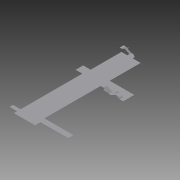
# Autodesk Inventor part: LabVIEWM0.5
Saved by Autodesk Inventor 2013 SP2 (Build 170200200, 200)
## iProperties
Created: 2014-11-17
Part Number: LabVIEWM0.5
Material: 常规
Document SubType Name: Modeling
Designer: 振胜
Density: 1 g/cm^3
Author: 振胜
Autodesk Inventor part; units mm, degrees
ref_plane "YZ Plane" through (0, 0, 0) normal (1, 0, 0) x (0, 1, 0)
sketch "DOOR" plane through (0, 0, 0) normal (0, 0, 1) x (1, 0, 0)
  line L0 (72.1652, -32.5468) -> (92.1652, -32.5468)
  line L1 (92.1652, -32.5468) -> (92.1652, -42.5468)
  line L2 (92.1652, -42.5468) -> (72.1652, -42.5468)
  line L3 (72.1652, -42.5468) -> (72.1652, -32.5468)
  line L4 (72.1652, -37.5468) -> (92.1652, -37.5468) construction
  dimension "d217" = 10
  dimension "d219" = 20
  measures "d217" distance between parallel lines of L2 L0
  measures "d219" distance between parallel lines of L1 L3
sketch "DOOR2" plane through (0, 0, 0) normal (0, 0, 1) x (1, 0, 0)
  line L0 (57.8646, 97.8913) -> (77.8646, 97.8913)
  line L1 (77.8646, 97.8913) -> (77.8646, 87.8913)
  line L2 (77.8646, 87.8913) -> (57.8646, 87.8913)
  line L3 (57.8646, 87.8913) -> (57.8646, 97.8913)
  line L4 (57.8646, 92.8913) -> (77.8646, 92.8913) construction
  dimension "d227" = 10
  dimension "d229" = 20
  measures "d227" distance between parallel lines of L2 L0
  measures "d229" distance between parallel lines of L1 L3
ref_plane "工作平面1" through (0, 0, 0) normal (0, 0, 1) x (1, 0, 0)
sketch "草图1" plane through (0, 0, 0) normal (0, 0, 1) x (1, 0, 0)
  line L0 (0, 0) -> (60, 0)
  line L1 (60, 0) -> (60, -1169.8)
  line L2 (60, -1169.8) -> (0, -1169.8)
  line L3 (0, -1169.8) -> (0, 0)
  line L4 (0, -80.6) -> (60, -80.6)
  line L5 (0, -191.9) -> (60, -191.9)
  line L6 (0, -276.5) -> (60, -276.5)
  line L7 (0, -335.9) -> (60, -335.9)
  line L8 (0, -420.6) -> (60, -420.6)
  line L9 (0, -550.6) -> (60, -550.6)
  line L10 (0, -677.8) -> (60, -677.8)
  line L11 (0, -782.9) -> (60, -782.9)
  line L12 (0, -839.5) -> (60, -839.5)
  line L13 (0, -923.6) -> (60, -923.6)
  line L14 (0, -1007.7) -> (60, -1007.7)
  line L15 (0, -1091.2) -> (60, -1091.2)
  line L16 (60, 0) -> (118.4, 0)
  line L17 (118.4, 0) -> (118.4, -23.7)
  line L18 (118.4, -23.7) -> (83.4, -23.7)
  line L19 (83.4, -23.7) -> (83.4, -79.7)
  line L20 (83.4, -79.7) -> (118.4, -79.7)
  line L21 (118.4, -79.7) -> (118.4, -137.6)
  line L22 (118.4, -137.6) -> (83.4, -137.6)
  line L23 (83.4, -137.6) -> (83.4, -276.5)
  line L24 (83.4, -276.5) -> (142.9, -276.5)
  line L25 (142.9, -276.5) -> (142.9, -379.5)
  line L26 (83.4, -276.5) -> (83.4, -379.5)
  line L27 (83.4, -379.5) -> (142.9, -379.5)
  line L28 (142.9, -379.5) -> (142.9, -463)
  line L29 (142.9, -463) -> (83.4, -463)
  line L30 (83.4, -463) -> (83.4, -379.5)
  line L31 (142.9, -463) -> (142.9, -566.2)
  line L32 (142.9, -566.2) -> (83.4, -566.2)
  line L33 (83.4, -566.2) -> (83.4, -463)
  line L34 (142.9, -566.2) -> (146.7, -566.2)
  line L35 (146.7, -566.2) -> (146.7, -616.2)
  line L36 (146.7, -616.2) -> (192.5, -616.2)
  line L37 (192.5, -616.2) -> (192.5, -673.2)
  line L38 (192.5, -616.2) -> (342.5, -616.2)
  line L39 (342.5, -616.2) -> (342.5, -673.2)
  line L40 (342.5, -673.2) -> (143.4, -673.2)
  line L41 (143.4, -673.2) -> (83.4, -673.2)
  line L42 (83.4, -673.2) -> (83.4, -1092.3)
  line L43 (83.4, -1092.3) -> (143.4, -1092.3)
  line L44 (143.4, -1092.3) -> (143.4, -673.2)
  line L45 (83.4, -754.3) -> (143.4, -754.3)
  line L46 (143.4, -837.8) -> (83.4, -837.8)
  line L47 (83.4, -893.6) -> (143.4, -893.6)
  line L48 (143.4, -978.3) -> (83.4, -978.3)
  line L49 (60, -1169.8) -> (188.1, -1169.8)
  line L50 (188.1, -1169.8) -> (188.1, -1092.3)
  line L51 (188.1, -1092.3) -> (143.4, -1092.3)
  line L52 (83.4, -1092.3) -> (83.4, -1117.3)
  line L53 (83.4, -1117.3) -> (188.1, -1117.3)
  line L54 (98.6, -1092.3) -> (98.6, -1117.3)
  line L55 (114.5, -1092.3) -> (114.5, -1117.3)
  line L56 (143.4, -1092.3) -> (143.4, -1117.3)
  line L57 (166.2, -1092.3) -> (166.2, -1117.3)
  line L58 (188.1, -1163.6) -> (336, -1163.6)
  line L59 (188.1, -1137.1) -> (336, -1137.1)
  line L60 (336, -1137.1) -> (336, -1163.6)
  line L61 (342.5, -616.2) -> (398.5, -616.2)
  line L62 (342.5, -673.2) -> (393, -673.2)
  line L63 (393, -673.2) -> (393, -1136.7)
  line L64 (393, -1136.7) -> (393, -1141.7)
  line L65 (393, -1136.7) -> (336, -1137.1)
  line L66 (336, -1163.6) -> (393, -1163.6)
  line L67 (393, -1163.6) -> (393, -1158.6)
  line L68 (393, -1163.6) -> (393, -1188.1)
  line L69 (393, -1188.1) -> (417, -1188.1)
  line L70 (417, -1188.1) -> (553.5, -1188.1)
  line L71 (542.5, -1023) -> (542.5, -911)
  line L72 (542.5, -911) -> (542.5, -800.2)
  line L73 (542.5, -800.2) -> (542.5, -673.6)
  line L74 (398.5, -499.2) -> (398.5, -384.2)
  line L75 (398.5, -616.2) -> (398.5, -499.2)
  line L76 (398.5, -616.2) -> (458.5, -616.2)
  line L77 (458.5, -616.2) -> (458.5, -384.2)
  line L78 (458.5, -384.2) -> (398.5, -384.2)
  line L79 (398.5, -499.2) -> (458.5, -499.2)
  line L80 (398.5, -441.7) -> (458.5, -441.7)
  line L81 (458.5, -384.2) -> (458.5, -354.2)
  line L82 (458.5, -354.2) -> (482.5, -369.2)
  line L83 (482.5, -369.2) -> (482.5, -384.2)
  line L84 (482.5, -384.2) -> (542.5, -384.2)
  line L85 (542.5, -384.2) -> (542.5, -413.6)
  line L86 (542.5, -413.6) -> (542.5, -443.7)
  line L87 (542.5, -443.7) -> (542.5, -498.7)
  line L88 (542.5, -498.7) -> (542.5, -616.2)
  line L89 (542.5, -413.6) -> (501.5, -413.6)
  line L90 (542.5, -443.7) -> (482.5, -443.7)
  line L91 (542.5, -616.2) -> (482.5, -616.2)
  line L92 (542.5, -498.7) -> (482.5, -498.7)
  line L93 (482.5, -410.1) -> (501.5, -410.1)
  line L94 (501.5, -410.1) -> (501.5, -423.1)
  line L95 (501.5, -423.1) -> (482.5, -423.1)
  line L96 (482.5, -384.2) -> (482.5, -410.1)
  line L97 (482.5, -423.1) -> (482.5, -616.2)
  line L98 (542.5, -616.2) -> (727.5, -616.2)
  line L99 (727.5, -616.2) -> (727.5, -673.6)
  line L100 (727.5, -673.6) -> (542.5, -673.6)
  line L101 (578, -673.6) -> (578, -726.6)
  line L102 (578, -726.6) -> (605, -726.6)
  line L103 (605, -726.6) -> (605, -673.6)
  line L104 (727.5, -673.6) -> (727.5, -726.6)
  line L105 (727.5, -726.6) -> (700.5, -726.6)
  line L106 (700.5, -726.6) -> (700.5, -673.6)
  line L107 (442.5, -384.2) -> (442.5, -354.2)
  line L108 (442.5, -354.2) -> (458.5, -354.2)
  line L109 (398.5, -384.2) -> (384.5, -384.2)
  line L110 (384.5, -384.2) -> (384.5, -354.2)
  line L111 (384.5, -354.2) -> (400.5, -354.2)
  line L112 (400.5, -354.2) -> (400.5, -384.2)
  line L113 (458.5, -673.3753) -> (458.5, -1136.7)
  line L114 (482.5, -673.4395) -> (482.5, -1136.7)
  line L115 (542.5, -673.6) -> (482.5, -673.4395)
  line L116 (458.5, -673.3753) -> (393, -673.2)
  line L117 (458.5, -673.3753) -> (483.6773, -673.4426) construction
  line L118 (393, -1136.7) -> (458.5, -1136.7)
  line L119 (482.5, -1136.7) -> (535.5, -1136.7)
  line L120 (458.5, -1136.7) -> (482.5, -1136.7) construction
  line L121 (542.5, -1136.7) -> (542.5, -1106.6) construction
  line L122 (553.5, -1188.1) -> (553.5, -1147.6)
  line L123 (553.5, -1147.6) -> (761.5, -1147.6)
  line L124 (761.5, -1147.6) -> (761.5, -1106.6)
  line L125 (761.5, -1106.6) -> (542.5, -1106.6)
  line L126 (535.5, -1106.6) -> (535.5, -1136.7)
  line L127 (542.5, -1106.6) -> (542.5, -1023)
  line L128 (535.5, -1136.7) -> (542.5, -1136.7) construction
  line L129 (542.5, -1106.6) -> (535.5, -1106.6)
  line L130 (542.5, -800.2) -> (482.5, -800.2)
  line L131 (542.5, -911) -> (482.5, -911)
  line L132 (542.5, -1023) -> (482.5, -1023)
  line L133 (458.5, -800.2) -> (393, -800.2)
  line L134 (482.5, -800.2) -> (458.5, -800.2) construction
  line L135 (458.5, -911) -> (393, -911)
  line L136 (482.5, -911) -> (458.5, -911) construction
  line L137 (458.5, -1023) -> (393, -1023)
  line L138 (482.5, -1023) -> (458.5, -1023) construction
  dimension "d1" = 60
  dimension "d2" = 80.6
  dimension "d3" = 111.3
  dimension "d4" = 84.6
  dimension "d5" = 59.4
  dimension "d6" = 84.7
  dimension "d7" = 130
  dimension "d8" = 127.2
  dimension "d9" = 105.1
  dimension "d10" = 56.6
  dimension "d11" = 84.1
  dimension "d12" = 84.1
  dimension "d13" = 83.5
  dimension "d14" = 78.6
  dimension "d15" = 58.4
  dimension "d16" = 23.7
  dimension "d17" = 35
  dimension "d18" = 56
  dimension "d19" = 57.9
  dimension "d20" = 35
  dimension "d21" = 138.9
  dimension "d22" = 59.5
  dimension "d23" = 103
  dimension "d24" = 83.5
  dimension "d25" = 103.2
  dimension "d26" = 59.5
  dimension "d27" = 3.8
  dimension "d28" = 50
  dimension "d29" = 45.8
  dimension "d30" = 57
  dimension "d31" = 150
  dimension "d32" = 57
  dimension "d33" = 199.1
  dimension "d34" = 60
  dimension "d36" = 81.1
  dimension "d37" = 83.5
  dimension "d38" = 55.8
  dimension "d39" = 84.7
  dimension "d40" = 114
  dimension "d41" = 128.1
  dimension "d42" = 25
  dimension "d43" = 15.2
  dimension "d44" = 15.9
  dimension "d45" = 28.9
  dimension "d46" = 22.8
  dimension "d47" = 21.9
  dimension "d48" = 147.9
  dimension "d49" = 6.2
  dimension "d50" = 26.5
  dimension "d51" = 56
  dimension "d52" = 50.5
  dimension "d53" = 463.5
  dimension "d54" = 5
  dimension "d55" = 5
  dimension "d56" = 24.5
  dimension "d57" = 24
  dimension "d58" = 136.5
  dimension "d60" = 112
  dimension "d61" = 110.8
  dimension "d62" = 126.6
  dimension "d64" = 117
  dimension "d65" = 115
  dimension "d66" = 60
  dimension "d67" = 30
  constraints: 274 end point, 81 perpendicular, 42 point on line, 25 parallel, 18 horizontal, 15 collinear, 4 vertical, 1 horizontal alignment, 1 midpoint, 1 vertical alignment, 30 other
  measures "d1" distance of L0.start L0.end
  measures "d2" distance between parallel lines of L4 L0
  measures "d3" distance between parallel lines of L5 L4
  measures "d4" distance between parallel lines of L6 L5
  measures "d5" distance between parallel lines of L7 L6
  measures "d6" distance between parallel lines of L8 L7
  measures "d7" distance between parallel lines of L9 L8
  measures "d8" distance between parallel lines of L10 L9
  measures "d9" distance between parallel lines of L11 L10
  measures "d10" distance between parallel lines of L12 L11
  measures "d11" distance between parallel lines of L13 L12
  measures "d12" distance between parallel lines of L14 L13
  measures "d13" distance between parallel lines of L15 L14
  measures "d14" distance between parallel lines of L2 L15
  measures "d15" distance of L0.end L16.end
  measures "d16" distance of L16.end L17.end
  measures "d17" distance of L17.end L18.end
  measures "d18" distance of L18.end L19.end
  measures "d19" distance of L20.end L21.end
  measures "d20" distance of L21.end L22.end
  measures "d21" distance of L22.end L23.end
  measures "d22" distance of L23.end L24.end
  measures "d23" distance of L24.end L25.end
  measures "d24" distance of L25.end L28.end
  measures "d25" distance of L28.end L31.end
  measures "d26" distance of L31.end L32.end
  measures "d27" distance of L31.end L34.end
  measures "d28" distance of L34.end L35.end
  measures "d29" distance of L35.end L36.end
  measures "d30" distance of L36.end L37.end
  measures "d31" distance of L36.end L38.end
  measures "d32" distance of L38.end L39.end
  measures "d33" distance of L39.end L40.end
  measures "d34" distance of L40.end L41.end
  measures "d36" distance between parallel lines of L45 L41
  measures "d37" distance between parallel lines of L46 L45
  measures "d38" distance between parallel lines of L47 L46
  measures "d39" distance between parallel lines of L48 L47
  measures "d40" distance between parallel lines of L43 L48
  measures "d41" distance of L2.start L49.end
  measures "d42" distance between parallel lines of L53 L51
  measures "d43" distance between parallel lines of L54 L52
  measures "d44" distance between parallel lines of L55 L54
  measures "d45" distance between parallel lines of L56 L55
  measures "d46" distance between parallel lines of L57 L56
  measures "d47" distance between parallel lines of L50 L57
  measures "d48" distance of L58.start L58.end
  measures "d49" distance between parallel lines of L49 L58
  measures "d50" distance between parallel lines of L58 L59
  measures "d51" distance of L38.end L61.end
  measures "d52" distance of L39.end L62.end
  measures "d53" distance of L62.end L63.end
  measures "d54" distance of L63.end L64.end
  measures "d55" distance of L66.end L67.end
  measures "d56" distance of L66.end L68.end
  measures "d57" distance of L68.end L69.end
  measures "d58" distance of L69.end L70.end
  measures "d60" distance of L71.start L71.end
  measures "d61" distance of L71.end L72.end
  measures "d62" distance of L72.end L73.end
  measures "d64" distance of L61.end L74.start
  measures "d65" distance of L74.start L74.end
  measures "d66" distance of L61.end L76.end
  measures "d67" distance of L77.end L81.end
surface extrude "拉伸曲面1" sketch "草图1" along normal blind 35 shown no curves L81 L82 L83
surface extrude "拉伸曲面2" sketch "草图1" along normal blind 35 shown no curves L84 L85
surface extrude "拉伸曲面3" sketch "草图1" along normal blind 35 shown no curves L78
surface extrude "拉伸曲面4" sketch "草图1" along normal blind 35 shown no curves L74
surface extrude "拉伸曲面5" sketch "草图1" along normal blind 35 shown no curves L76 L77
surface extrude "拉伸曲面6" sketch "草图1" along normal blind 35 shown no curves L75
surface extrude "拉伸曲面7" sketch "草图1" along normal blind 35 shown no curves L80
surface extrude "拉伸曲面8" sketch "草图1" along normal blind 35 shown no curves L79
surface extrude "拉伸曲面9" sketch "草图1" along normal blind 35 shown no curves L96 L93 L94 L95 L97 L91
surface extrude "拉伸曲面10" sketch "草图1" along normal blind 35 shown no curves L89
surface extrude "拉伸曲面11" sketch "草图1" along normal blind 35 shown no curves L90
surface extrude "拉伸曲面12" sketch "草图1" along normal blind 35 shown no curves L86
surface extrude "拉伸曲面13" sketch "草图1" along normal blind 35 shown no curves L87
surface extrude "拉伸曲面14" sketch "草图1" along normal blind 35 shown no curves L92
surface extrude "拉伸曲面15" sketch "草图1" along normal blind 35 shown no curves L88
surface extrude "拉伸曲面16" sketch "草图1" along normal blind 35 shown no curves L61
surface extrude "拉伸曲面17" sketch "草图1" along normal blind 35 shown no curves L62
surface extrude "拉伸曲面18" sketch "草图1" along normal blind 35 shown no curves L115 L114 L119 L126 L129
surface extrude "拉伸曲面23" sketch "草图1" along normal blind 35 shown no curves L68 L69 L70 L122 L123 L124 L125
surface extrude "拉伸曲面25" sketch "草图1" along normal blind 35 shown no curves L71
surface extrude "拉伸曲面27" sketch "草图1" along normal blind 35 shown no curves L72
surface extrude "拉伸曲面29" sketch "草图1" along normal blind 35 shown no curves L73
extrude "拉伸5" add sketch "草图1" against normal blind 1 contours L60 L65 L118 L113 L116 L62 L39 L61 L76 L77 L81 L82 L83 L96 L93 L94 L95 L97 L91 L98 L99 L100 L115 L114 L119 L126 L129 L125 L124 L123 L122 L70 L69 L68 L66 | L75 L79 L77 L76 | L63 L137 L113 L118 | L116 L113 L133 L63 | L74 L80 L77 L79 | L63 L135 L113 L137 | L133 L113 L135 L63 | L74 L78 L77 L80 | L109 L110 L111 L112 L78 | L78 L107 L108 L81 | L129 L126 L119 L114 L132 L127 | L84 L85 L89 L94 L93 L96 | L132 L114 L131 L71 | L131 L114 L130 L72 | L86 L90 L97 L95 L94 L89 | L130 L114 L115 L73 | L87 L92 L97 L90 | L88 L91 L97 L92 | L100 L103 L102 L101 | L100 L104 L105 L106
ref_plane "工作平面8" through (442.5, -369.2, 0) normal (0, 1, 0) x (1, 0, 0)
sketch "草图6" plane through (442.5, -369.2, 0) normal (0, 1, 0) x (1, 0, 0)
  line L0 (0, 0) -> (0, 1) construction
  line L1 (0, 0.5) -> (-42, -20.5)
  line L2 (0, 0.5) -> (0, 0.1)
  line L3 (0, 0.1) -> (-42, -20.9)
  line L4 (-42, -20.9) -> (-42, -20.5)
  line L5 (-42, -20.9) -> (-58, -20.9)
  line L6 (-58, -20.9) -> (-58, -20.5)
  line L7 (-58, -20.5) -> (-42, -20.5)
  point P0 (-442.5, 0)
  dimension "d258" = 42
  dimension "d260" = 21
  dimension "d261" = 0.4
  dimension "d262" = 16
  constraints: 14 end point, 2 parallel, 2 perpendicular, 1 horizontal, 1 midpoint, 1 point on line
  measures "d258" horizontal distance of L1.start L1.end
  measures "d260" vertical distance of L1.start L1.end
  measures "d261" distance of L1.start L2.end
  measures "d262" distance of L3.end L5.end
extrude "拉伸6" add sketch "草图6" along normal up to surface (15 mm away)
sketch "草图7" plane through (442.5, -369.2, 0) normal (0, -1, 0) x (1, 0, 0)
  line L0 (-58, 20.5) -> (-58, 20.9) construction
  line L1 (-58, 20.9) -> (-42, 20.9) construction
  line L2 (-42, 20.5) -> (-58, 20.5) construction
  line L3 (-58, 20.9) -> (-42, 20.9)
  line L4 (-42, 20.9) -> (-42, 20.5)
  line L5 (-42, 20.5) -> (-58, 20.5)
  line L6 (-58, 20.5) -> (-58, 20.9)
  line L7 (-42, 20.5) -> (0, 41.5)
  line L8 (-42, 20.9) -> (0, 41.9)
  line L9 (0, 41.9) -> (0, 41.5)
  point P0 (-442.5, 0)
  dimension "d265" = 21
  dimension "d266" = 42
  constraints: 14 end point, 3 parallel, 1 horizontal, 1 perpendicular, 1 vertical
  measures "d265" vertical distance of L2.start L7.end
  measures "d266" horizontal distance of L2.start L7.end
extrude "拉伸7" add sketch "草图7" along normal up to surface (15 mm away)
sketch "草图8" plane through (0, 0, -1) normal (0, 0, -1) x (-1, 0, 0)
  line L0 (-384.5, -354.2) -> (-384.5, -384.2) projected
  line L1 (-400.5, -354.2) -> (-384.5, -354.2) projected
  line L2 (-400.5, -384.2) -> (-400.5, -354.2) projected
  line L3 (-384.5, -384.2) -> (-400.5, -384.2)
  point P0 (0, 0)
  constraints: 2 end point, 1 perpendicular
extrude "拉伸8" cut sketch "草图8" against normal up to surface (1 mm away)
sketch "草图9" plane through (0, 0, 0) normal (0, 0, 1) x (1, 0, 0)
  line L0 (578, -673.6) -> (578, -726.6) construction
  line L1 (578, -726.6) -> (605, -726.6) construction
  line L2 (605, -726.6) -> (605, -673.6) construction
  line L3 (700.5, -673.6) -> (700.5, -726.6) construction
  line L4 (727.5, -726.6) -> (727.5, -616.2) construction
  line L5 (700.5, -726.6) -> (727.5, -726.6) construction
  line L6 (578, -726.6) -> (605, -726.6)
  line L7 (605, -726.6) -> (605, -700.1)
  line L8 (605, -700.1) -> (578, -700.1)
  line L9 (578, -700.1) -> (578, -726.6)
  line L10 (727.5, -726.6) -> (700.5, -726.6)
  line L11 (700.5, -726.6) -> (700.5, -700.1)
  line L12 (700.5, -700.1) -> (727.5, -700.1)
  line L13 (727.5, -700.1) -> (727.5, -726.6)
  point P0 (0, 0)
  constraints: 16 end point, 4 parallel, 2 horizontal, 2 midpoint, 2 perpendicular
extrude "拉伸9" cut sketch "草图9" against normal blind 10
sketch "草图10" plane through (700.5, -700.1, 0) normal (0, -1, 0) x (1, 0, 0)
  line L0 (0, -1) -> (0, 0) construction
  line L1 (-95.5, 0) -> (-95.5, -1) construction
  line L2 (0, -0.5) -> (-42, 20.5)
  line L3 (-95.5, -0.5) -> (-53.5, 20.5)
  line L4 (-95.5, -0.5) -> (-95.5, -0.1)
  line L5 (-95.5, -0.1) -> (-53.5, 20.9)
  line L6 (-53.5, 20.9) -> (-53.5, 20.5)
  line L7 (0, -0.5) -> (0, -0.1)
  line L8 (0, -0.1) -> (-42, 20.9)
  line L9 (-42, 20.9) -> (-42, 20.5)
  line L10 (-53.5, 20.9) -> (-42, 20.9)
  line L11 (-42, 20.5) -> (-53.5, 20.5)
  point P0 (-700.5, 0)
  dimension "d273" = 42
  dimension "d275" = 21
  dimension "d276" = 42
  dimension "d277" = 21
  dimension "d278" = 0.4
  dimension "d279" = 0.4
  constraints: 20 end point, 2 midpoint, 2 parallel, 2 point on line, 2 vertical
  measures "d273" horizontal distance of L3.start L3.end
  measures "d275" vertical distance of L3.start L3.end
  measures "d276" horizontal distance of L2.start L2.end
  measures "d277" vertical distance of L2.start L2.end
  measures "d278" distance of L3.start L4.end
  measures "d279" distance of L2.start L7.end
extrude "拉伸10" add sketch "草图10" against normal up to surface (26.5 mm away)
sketch "草图11" plane through (700.5, -700.1, 0) normal (0, -1, 0) x (1, 0, 0)
  line L0 (-42, 20.9) -> (-53.5, 20.9) construction
  line L1 (-53.5, 20.5) -> (-42, 20.5) construction
  line L2 (-53.5, 20.9) -> (-42, 20.9)
  line L3 (-42, 20.9) -> (-42, 20.5)
  line L4 (-42, 20.5) -> (-53.5, 20.5)
  line L5 (-53.5, 20.5) -> (-53.5, 20.9)
  line L6 (-53.5, 20.5) -> (-95.5, 41.5)
  line L7 (-42, 20.5) -> (0, 41.5)
  line L8 (-53.5, 20.9) -> (-95.5, 41.9)
  line L9 (-95.5, 41.9) -> (-95.5, 41.5)
  line L10 (-42, 20.9) -> (0, 41.9)
  line L11 (0, 41.9) -> (0, 41.5)
  line L12 (0, 41.9) -> (27, 41.9)
  line L13 (27, 41.9) -> (27, 41.5)
  line L14 (27, 41.5) -> (0, 41.5)
  line L15 (-95.5, 41.9) -> (-122.5, 41.9)
  line L16 (-122.5, 41.9) -> (-122.5, 41.5)
  line L17 (-122.5, 41.5) -> (-95.5, 41.5)
  point P0 (-700.5, 0)
  dimension "d282" = 42
  dimension "d284" = 42
  dimension "d285" = 21
  dimension "d286" = 21
  dimension "d289" = 27
  dimension "d290" = 0.4
  dimension "d291" = 27
  dimension "d292" = 0.4
  constraints: 32 end point, 5 parallel, 4 perpendicular, 2 vertical, 1 horizontal
  measures "d282" horizontal distance of L4.end L6.end
  measures "d284" horizontal distance of L1.end L7.end
  measures "d285" vertical distance of L1.end L7.end
  measures "d286" vertical distance of L4.end L6.end
  measures "d289" distance of L10.end L12.end
  measures "d290" distance of L12.end L13.end
  measures "d291" distance of L8.end L15.end
  measures "d292" distance of L15.end L16.end
extrude "拉伸11" add sketch "草图11" along normal blind 26.5
